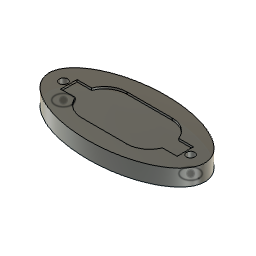
foreo (Autodesk Fusion 360 design; units mm, degrees)
Autodesk Fusion 360 part; units mm, degrees
note: some values were not read from the file. Set by a fixed rule: which sketch regions a step uses.
sketch "Sketch1" plane through (0, 0, 0) normal (0, 0, 1) x (1, 0, 0)
  line L0 (0, 0) -> (19, 0)
  line L1 (0, 0) -> (-19, 0)
  spline S0 degree 5 poles (-19, 0) (-19, 0.5932) (-18.8095, 1.7795) (-17.9524, 3.5307) (-15.714, 5.6956) (-11.3912, 7.857) (-5.9789, 9.256) (0, 9.742) (5.9789, 9.256) (11.3912, 7.857) (15.714, 5.6956) (18.512, 2.9894) (19.484, 0) (18.512, -2.9894) (15.714, -5.6956) (11.3912, -7.857) (5.9789, -9.256) (0, -9.742) (-5.9789, -9.256) (-11.3912, -7.857) (-15.714, -5.6956) (-17.9524, -3.5307) (-18.8095, -1.7795) (-19, -0.5932) (-19, 0) knots 0 0 0 0 0 0 0.05 0.1 0.15 0.2 0.25 0.3 0.35 0.4 0.45 0.5 0.55 0.6 0.65 0.7 0.75 0.8 0.85 0.9 0.95 1 1 1 1 1 1
  line L2 (0, 0) -> (-5.5, 0)
  circle A0 centre (-5.5, 0) radius 5.5
  line L3 (0, 0) -> (5.5, 0)
  circle A1 centre (5.5, 0) radius 5.5
  line L4 (-5.5, 5.5) -> (5.5, 5.5)
  line L5 (-5.5, -5.5) -> (5.5, -5.5)
  line L6 (-11, 0) -> (-15.5, 0)
  line L7 (11, 0) -> (15.5, 0)
  circle A2 centre (-15.5, 0) radius 1
  circle A3 centre (15.5, 0) radius 1
  line L8 (-14.1915, 1.5) -> (-14.1915, -1.5)
  line L9 (14.1915, 1.5) -> (14.1915, -1.5)
  line L10 (-10, -2) -> (-14.1915, -2)
  line L11 (-14.1915, -2) -> (-14.1915, 2)
  line L12 (-14.1915, 2) -> (-10, 2)
  line L13 (10, 2) -> (14.198, 2)
  line L14 (14.198, 2) -> (14.198, -2)
  line L15 (14.198, -2) -> (10, -2)
  point P0 (0, 9.5)
  point P1 (0, -9.5)
  dimension "d1" = 19
  dimension "d2" = 19
  dimension "d3" = 9.5
  dimension "d4" = 9.5
  dimension "d5" = 5.5
  dimension "d6" = 5.5
  dimension "d7" = 11
  dimension "d8" = 4.5
  dimension "d9" = 4.5
  dimension "d10" = 2
  dimension "d11" = 2
  constraint coincident L0.start L1.start
  constraint horizontal L0
  constraint parallel L0 L1
  constraint coincident L2.end A0.centre
  constraint coincident L0.start A0
  constraint coincident L3.end A1.centre
  constraint coincident A0 L4.start
  constraint coincident A1 L4.end
  constraint tangent A1 L4
  constraint coincident A0 L5.start
  constraint coincident A1 L5.end
  constraint tangent A1 L5
  constraint coincident A0 L6.start
  constraint coincident L1 L6.start
  constraint parallel L1 L6
  constraint coincident L0 L7.start
  constraint coincident A1 L7.start
  constraint parallel L0 L7
  constraint coincident L6.end A2.centre
  constraint coincident L7.end A3.centre
  constraint perpendicular L8 L10
  constraint perpendicular L14 L15
  measures "d1" distance of L0.start L0.end
  measures "d2" distance of L0.start L1.end
  measures "d3" distance of L0.start P0
  measures "d4" distance of L0.start P1
  measures "d5" distance of L0.start L2.end
  measures "d6" distance of L0.start L3.end
  measures "d7" diameter of A1
  measures "d8" distance of L6.start L6.end
  measures "d9" distance of L7.start L7.end
  measures "d10" diameter of A2
  measures "d11" diameter of A3
extrude "Extrude7" add sketch "Sketch1" along normal blind 4 contours L0 L1 S0 A0 A1 L4 L6 L7 A2 A3 L8 L11 L12 L13 L14 | L0 L1 S0 A0 A1 L5 L6 L7 A2 A3 L8 L10 L11 L14 L15
extrude "Extrude8" add sketch "Sketch1" along normal blind 3.5 contours L0 L3 A1 | L1 L2 A0 | L1 L2 A0 | A0 A1 L5 | A0 A1 L4 | L0 L3 A1 | L0 A1 L7 L13 L14 | L0 A1 L7 L14 L15 | L1 A0 L6 L8 L10 L11 | L1 A0 L6 L8 L11 L12
sketch "Sketch2" plane through (0, 0, 0) normal (0, 0, -1) x (1, 0, 0)
  circle A0 centre (15.5, 0) radius 1
  circle A1 centre (-15.5, 0) radius 1
  spline S0 degree 5 poles (-19, 0) (-19, -0.5932) (-18.8095, -1.7795) (-17.9524, -3.5307) (-15.714, -5.6956) (-11.3912, -7.857) (-5.9789, -9.256) (0, -9.742) (5.9789, -9.256) (11.3912, -7.857) (15.714, -5.6956) (18.512, -2.9894) (19.484, 0) (18.512, 2.9894) (15.714, 5.6956) (11.3912, 7.857) (5.9789, 9.256) (0, 9.742) (-5.9789, 9.256) (-11.3912, 7.857) (-15.714, 5.6956) (-17.9524, 3.5307) (-18.8095, 1.7795) (-19, 0.5932) (-19, 0) knots 0 0 0 0 0 0 0.05 0.1 0.15 0.2 0.25 0.3 0.35 0.4 0.45 0.5 0.55 0.6 0.65 0.7 0.75 0.8 0.85 0.9 0.95 1 1 1 1 1 1
  circle A2 centre (-15.5, 0) radius 2
  circle A3 centre (15.5, 0) radius 2
  dimension "d36" = 4
  dimension "d37" = 4
  constraint concentric A1 A2
  constraint concentric A0 A3
  measures "d36" diameter of A2
  measures "d37" diameter of A3
extrude "Extrude9" cut sketch "Sketch2" against normal blind 2 contours A2
extrude "Extrude10" cut sketch "Sketch2" against normal blind 2 contours A3
